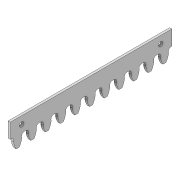
# Autodesk Inventor part: rack
Saved by Autodesk Inventor 2020 (Build 240168000, 168)
## iProperties
Created: 2021-06-14
Part Number: rack
Material: Generic
Document SubType Name: Modeling
Designer: Aidan Lee
Density: 1 g/cm^3
Appearance: Default
Author: Aidan Lee
Autodesk Inventor part; units mm, degrees
ref_plane "YZ Plane" through (0, 0, 0) normal (1, 0, 0) x (0, 1, 0)
ref_plane "XZ Plane" through (0, 0, 0) normal (0, 1, 0) x (-1, 0, 0)
ref_plane "XY Plane" through (0, 0, 0) normal (0, 0, 1) x (1, 0, 0)
sketch "Sketch2" plane through (0, 0, 0) normal (0, 0, 1) x (1, 0, 0)
  line L0 (-32.0857, 0) -> (0, 0)
  line L1 (0, 0) -> (0, 19.635)
  line L2 (0, 19.635) -> (-32.0857, 19.635)
  spline S0 degree 3 poles (-32.0857, 19.635) (-32.0786, 19.6019) (-32.0585, 19.4984) (-32.0378, 19.3226) (-32.0222, 19.1083) (-32.0293, 18.8935) (-32.0484, 18.6795) (-32.102, 18.3981) (-32.1765, 18.0482) (-32.2416, 17.6965) (-32.2997, 17.416) (-32.364, 17.211) (-32.4396, 17.0099) (-32.536, 16.8179) (-32.6409, 16.6304) (-32.7641, 16.4543) (-32.8983, 16.2866) (-33.043, 16.1278) (-33.201, 15.9822) (-33.3669, 15.8459) (-33.5414, 15.7205) (-33.7857, 15.5713) (-34.1055, 15.4094) (-34.509, 15.2608) (-34.9249, 15.1525) (-35.3479, 15.078) (-35.7753, 15.0341) (-36.2047, 15.0215) (-36.6341, 15.0313) (-37.0623, 15.0646) (-37.3462, 15.1014) (-37.4881, 15.1198) knots -0.847201 -0.847201 -0.847201 -0.847201 -0.83705 -0.815587 -0.794126 -0.772659 -0.751201 -0.729734 -0.686802 -0.64387 -0.622403 -0.600945 -0.579478 -0.558017 -0.536554 -0.515088 -0.49363 -0.472163 -0.450698 -0.429238 -0.407769 -0.386302 -0.343394 -0.300476 -0.257562 -0.214646 -0.17172 -0.12879 -0.085861 -0.04293 0 0 0 0
  spline S1 degree 3 poles (-37.4881, 15.1198) (-37.594, 15.1249) (-37.8057, 15.1352) (-38.2295, 15.119) (-38.7575, 15.0717) (-39.3865, 14.9771) (-40.0103, 14.8535) (-40.6285, 14.7043) (-41.2408, 14.5326) (-41.847, 14.3405) (-42.4469, 14.1297) (-43.0405, 13.9015) (-43.6276, 13.6572) (-44.2081, 13.3977) (-44.782, 13.1239) (-45.3493, 12.8367) (-45.9097, 12.5363) (-46.4639, 12.2246) (-46.8275, 12.0066) (-47.0092, 11.8976) knots -1.017256 -1.017256 -1.017256 -1.017256 -0.985476 -0.953687 -0.890117 -0.826542 -0.762964 -0.699386 -0.635807 -0.572227 -0.508647 -0.445066 -0.381486 -0.317905 -0.254324 -0.190743 -0.127162 -0.063581 0 0 0 0
  arc A0 (-47.0092, 11.8976) -> (-47.0092, 7.7374) centre (9.2023, 9.8175) ccw
  spline S2 degree 3 poles (-47.0092, 7.7374) (-46.8275, 7.6284) (-46.4639, 7.4104) (-45.9097, 7.0987) (-45.3493, 6.7983) (-44.782, 6.5111) (-44.2081, 6.2373) (-43.6276, 5.9778) (-43.0405, 5.7335) (-42.4469, 5.5053) (-41.847, 5.2945) (-41.2408, 5.1024) (-40.6285, 4.9307) (-40.0103, 4.7815) (-39.3865, 4.6579) (-38.7575, 4.5633) (-38.2295, 4.516) (-37.8057, 4.4998) (-37.594, 4.5101) (-37.4881, 4.5152) knots -1.017256 -1.017256 -1.017256 -1.017256 -0.953675 -0.890094 -0.826513 -0.762932 -0.699351 -0.63577 -0.572189 -0.508609 -0.445029 -0.381449 -0.31787 -0.254291 -0.190714 -0.127139 -0.063568 -0.03178 0 0 0 0
  spline S3 degree 3 poles (-37.4881, 4.5152) (-37.3462, 4.5336) (-37.0623, 4.5704) (-36.6341, 4.6037) (-36.2047, 4.6135) (-35.7753, 4.6009) (-35.3479, 4.557) (-34.9249, 4.4825) (-34.509, 4.3742) (-34.1055, 4.2256) (-33.7857, 4.0637) (-33.5414, 3.9145) (-33.3669, 3.7891) (-33.201, 3.6528) (-33.043, 3.5072) (-32.8983, 3.3484) (-32.7641, 3.1807) (-32.6409, 3.0046) (-32.536, 2.8171) (-32.4396, 2.6251) (-32.364, 2.424) (-32.2997, 2.219) (-32.2416, 1.9385) (-32.1765, 1.5868) (-32.102, 1.2369) (-32.0484, 0.9555) (-32.0293, 0.7415) (-32.0222, 0.5267) (-32.0378, 0.3124) (-32.0585, 0.1366) (-32.0786, 0.0331) (-32.0857, 0) knots -1.373604 -1.373604 -1.373604 -1.373604 -1.330674 -1.287743 -1.244814 -1.201884 -1.158958 -1.116042 -1.073128 -1.03021 -0.987302 -0.965835 -0.944366 -0.922906 -0.901441 -0.879974 -0.858516 -0.83705 -0.815587 -0.794126 -0.772659 -0.751201 -0.729734 -0.686802 -0.64387 -0.622403 -0.600945 -0.579478 -0.558017 -0.536554 -0.526403 -0.526403 -0.526403 -0.526403
  constraints: 6 end point, 2 centre point, 2 point on circle, 16 other
extrude "Extrusion1" add sketch "Sketch2" along normal blind 3
pattern_linear "Rectangular Pattern1" count 11 spacing 19.635 along (0, 1, 0) of "Extrusion1"
sketch "Sketch4" plane through (0, 0, 0) normal (0, 0, -1) x (-1, 0, 0)
  line L0 (32.0857, 0) -> (0, 0) projected
  line L1 (0, 0) -> (0, 215.985) projected
  line L2 (0, 215.985) -> (32.0857, 215.985) projected
  line L3 (0, 0) -> (12.0857, 0)
  line L4 (12.0857, 0) -> (12.0857, 215.985)
  line L5 (12.0857, 215.985) -> (0, 215.985)
  line L6 (0, 215.985) -> (0, 0)
  circle A0 centre (22.0857, 15) radius 3
  line L7 (-30.0969, 107.9925) -> (-14.6902, 107.9925) construction
  circle A1 centre (22.0857, 200.985) radius 3
  point P0 (0, 107.9925)
  point P1 (-22.3936, 107.9925)
  dimension "d6" = 32.0857
  dimension "d7" = 20
  dimension "d8" = 6
  dimension "d10" = 10
  dimension "d11" = 15
  constraints: 10 end point, 2 centre point, 2 horizontal, 2 midpoint, 2 parallel, 1 horizontal alignment, 1 perpendicular, 1 point on line, 1 symmetric about line, 1 other
  measures "d6" distance of L0.start L0.end
  measures "d7" distance from line of L0.start L4
  measures "d8" diameter of A0
  measures "d10" distance from line of L4 A0.centre
  measures "d11" distance from line of L0 A0.centre
extrude "Extrusion2" cut sketch "Sketch4" against normal through all
body "Solid1"
